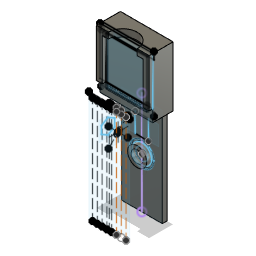
Variante Stifte Unten 20200217 v29 (Autodesk Fusion 360 archive; units mm, degrees)
design "Variante1"
Autodesk Fusion 360 part; units mm, degrees
mesh "Netz1" [no effect]
mesh "Netz2" [no effect]
sketch "Skizze1" plane through (0, 0, 0) normal (1, 0, 0) x (0, 0, -1)
  line L0 (1.7531, 23.1259) -> (1.7531, 20)
  line L1 (1.7531, 20) -> (-2.7469, 20)
  line L2 (-2.7469, 20) -> (-2.7469, -23)
  line L3 (-2.7469, -23) -> (-5.2469, -23)
  line L4 (-5.2469, -23) -> (-5.2469, 23.071)
  line L5 (1.7531, 23.071) -> (-5.2469, 23.071)
  dimension "d1" = 4.5
  dimension "d2" = 2.5
  dimension "d3" = 7.0002
  constraint vertical L0
  constraint perpendicular L0 L1
  constraint perpendicular L1 L2
  constraint perpendicular L2 L3
  constraint perpendicular L3 L4
  constraint coincident L0 L5.start
  constraint coincident L4 L5.end
  constraint perpendicular L4 L5
  measures "d1" distance of L0.end L1.end
  measures "d2" distance of L2.end L3.end
  measures "d3" distance of L0.start L4.end
extrude "Extrusion1" add sketch "Skizze1" along normal blind 8.5 makes body 1
extrude "Extrusion2" add 1 faces at (0, 22.0473, 2.0803) along direction (-1, 0, 0) blind 8.5 on bodies 1 bodies 1
sketch "Skizze2" plane through (0, 0, 2.7469) normal (0, 0, -1) x (-1, 0, 0)
  line L0 (8.5, 20) -> (-8.5, 20)
  line L1 (-8.5, 20) -> (-8.5, -23)
  line L2 (-8.5, -23) -> (8.5, -23)
  line L3 (8.5, -23) -> (8.5, 20)
  line L4 (2.8119, 12.0538) -> (-2.7881, 12.0538)
  line L5 (-2.7881, 12.0538) -> (-2.7881, 4.0538)
  line L6 (-2.7881, 4.0538) -> (2.8119, 4.0538)
  line L7 (2.8119, 4.0538) -> (2.8119, 12.0538)
  dimension "d8" = 5.6
  dimension "d9" = 8
  constraint horizontal L4
  constraint vertical L5
  constraint horizontal L6
  constraint vertical L7
  measures "d8" distance of L4.start L4.end
  measures "d9" distance of L4.start L6.end
extrude "Extrusion3" add sketch "Skizze2" along normal blind 8 contours L4 L5 L6 L7 bodies 1
sketch "Skizze3" plane through (-2.8119, 0, 0) normal (-1, 0, 0) x (0, 0, 1)
  line L0 (2.7469, 4.0538) -> (2.7469, 12.0538)
  line L1 (2.7469, 12.0538) -> (-5.2531, 12.0538)
  line L2 (-5.2531, 12.0538) -> (-5.2531, 4.0538)
  line L3 (-5.2531, 4.0538) -> (2.7469, 4.0538)
  line L4 (2.7469, 12.0538) -> (-5.2531, 4.0538) construction
  line L5 (2.7469, 4.0538) -> (-5.2531, 12.0538) construction
  circle A0 centre (-1.2531, 8.0538) radius 1.6
  line L6 (-5.2531, 8.0538) -> (-1.2531, 8.0538) construction
  line L7 (-1.2531, 8.0538) -> (2.7469, 8.0538) construction
  line L8 (-1.2531, 8.0538) -> (-1.2531, 12.0538) construction
  line L9 (-1.2531, 8.0538) -> (-1.2531, 4.0538) construction
  dimension "d12" = 3.2
  dimension "d13" = 8
  dimension "d14" = 8
  constraint coincident L0.end L1.start
  constraint coincident L2.end L3.start
  constraint coincident L0.start L3.end
  constraint coincident L1.end L2.start
  constraint midpoint L4 A0.centre
  constraint midpoint L2 L6.start
  constraint coincident A0.centre L6.end
  constraint midpoint L0 L7.end
  constraint midpoint L1 L8.end
  constraint midpoint L3 L9.end
  measures "d12" diameter of A0
  measures "d13" distance of L0 L2
  measures "d14" distance of L1.end L2.end
sketch "Skizze4" plane through (0, 0, 0) normal (1, 0, 0) x (0, 0, -1)
extrude "Extrusion4" add sketch "Skizze3" against normal blind 5.6 separate body makes body 2
sketch "Skizze5" plane through (0, 0, 2.7469) normal (0, 0, -1) x (-1, 0, 0)
  circle A0 centre (0, -1.9896) radius 2.4976 construction
  line L0 (0, 20) -> (0, -23) construction
  circle A1 centre (0, -1.9896) radius 2.5 construction
  circle A2 centre (0, -1.9896) radius 2.5
  circle A3 centre (0, -1.9896) radius 5
  circle A4 centre (0, -1.9896) radius 4
  dimension "d17" = 5
  dimension "d18" = 5
  dimension "d19" = 10
  dimension "d20" = 8
  constraint concentric A0 A1
  constraint concentric A1 A2
  constraint concentric A2 A3
  constraint concentric A1 A4
  measures "d17" diameter of A1
  measures "d18" diameter of A2
  measures "d19" diameter of A3
  measures "d20" diameter of A4
extrude "Extrusion5" add sketch "Skizze5" along normal blind 1 separate body contours A4 makes body 3
extrude "Extrusion6" add sketch "Skizze5" against normal blind 1 separate body contours A3 makes body 4
extrude "Extrusion7" cut sketch "Skizze5" against normal blind 1 contours A3 bodies 1 4
sketch "Skizze6" plane through (0, 0, 5.2469) normal (0, 0, 1) x (1, 0, 0)
  line L0 (-8.5, -23) -> (8.5, -23)
  line L1 (8.5, -23) -> (8.5, 23.071)
  line L2 (8.5, 23.071) -> (-8.5, 23.071)
  line L3 (-8.5, 23.071) -> (-8.5, -23)
  line L4 (-8.5, 23.071) -> (-8.5, 21.571) construction
  line L5 (-8.5, 21.571) -> (8.5, 21.571) construction
  line L6 (-8.5, 23.071) -> (0, 23.071) construction
  line L7 (0, 23.071) -> (0, -23) construction
  line L8 (0, 23.071) -> (1, 23.071) construction
  line L9 (1, 23.071) -> (3, 23.071) construction
  line L10 (3, 23.071) -> (5, 23.071) construction
  line L11 (0, 23.071) -> (-1, 23.071) construction
  line L12 (1, 23.071) -> (1, -23) construction
  line L13 (-1, 23.071) -> (-1, -23) construction
  line L14 (1, 23.071) -> (3, 23.071) construction
  line L15 (3, 23) -> (5, 23) construction
  line L16 (5, 23) -> (7, 23) construction
  line L17 (-1, 23.071) -> (-3, 23.071) construction
  line L18 (-3, 23.071) -> (-5, 23.071) construction
  line L19 (-5, 23.071) -> (-7, 23.071) construction
  line L20 (7, 23) -> (7, -23) construction
  line L21 (5, 23.071) -> (5, -23) construction
  line L22 (3, 23) -> (3, -23) construction
  line L23 (-3, 23.071) -> (-3, -23) construction
  line L24 (-5, 23.071) -> (-5, -23) construction
  line L25 (-7, 23.071) -> (-7, -23) construction
  circle A0 centre (7, 21.571) radius 0.5
  circle A1 centre (5, 21.571) radius 0.5
  circle A2 centre (3, 21.571) radius 0.5
  circle A3 centre (1, 21.571) radius 0.5
  circle A4 centre (-1, 21.571) radius 0.5
  circle A5 centre (-3, 21.571) radius 0.5
  circle A6 centre (-5, 21.571) radius 0.5
  circle A7 centre (-7, 21.571) radius 0.5
  point P0 (0, 23.071)
  dimension "d27" = 1.5
  dimension "d28" = 1
  dimension "d29" = 1
  dimension "d30" = 2
  dimension "d31" = 2
  dimension "d32" = 2
  dimension "d33" = 2
  dimension "d34" = 2
  dimension "d35" = 2
  dimension "d36" = 1
  dimension "d37" = 1
  dimension "d38" = 1
  dimension "d39" = 1
  dimension "d40" = 1
  dimension "d41" = 1
  dimension "d42" = 1
  dimension "d43" = 1
  constraint coincident L2.end L3.start
  constraint perpendicular L2 L4
  constraint coincident L1 L5.end
  constraint perpendicular L1 L5
  constraint coincident P0 L6.end
  constraint midpoint L0 L7.end
  constraint coincident L2 L8.end
  constraint coincident L2 L9.end
  constraint perpendicular L1 L9
  constraint coincident L2 L10.end
  constraint perpendicular L7 L11
  constraint coincident L0 L12.end
  constraint perpendicular L0 L12
  constraint coincident L0 L13.end
  constraint perpendicular L0 L13
  constraint perpendicular L12 L14
  constraint parallel L2 L15
  constraint parallel L15 L16
  constraint perpendicular L13 L17
  constraint parallel L2 L18
  constraint parallel L2 L19
  constraint coincident L0 L20.end
  constraint perpendicular L0 L20
  constraint perpendicular L10 L21
  constraint coincident L0 L22.end
  constraint perpendicular L0 L22
  constraint coincident L0 L23.end
  constraint perpendicular L0 L23
  constraint coincident L0 L24.end
  constraint perpendicular L0 L24
  constraint coincident L0 L25.end
  constraint perpendicular L0 L25
  constraint coincident L5 A0.centre
  constraint coincident L20 A0.centre
  constraint coincident L21 A1.centre
  constraint coincident L5 A1.centre
  constraint coincident L22 A2.centre
  constraint coincident L5 A2.centre
  constraint coincident L12 A3.centre
  constraint coincident L5 A3.centre
  constraint coincident L13 A4.centre
  constraint coincident L5 A4.centre
  constraint coincident L23 A5.centre
  constraint coincident L5 A5.centre
  constraint coincident L24 A6.centre
  constraint coincident L5 A6.centre
  constraint coincident L25 A7.centre
  constraint coincident L5 A7.centre
  measures "d27" distance of L2.end L4.end
  measures "d28" distance of P0 L8.end
  measures "d29" distance of P0 L11.end
  measures "d30" distance of L8.end L9.end
  measures "d31" distance of L15.start L15.end
  measures "d32" distance of L15.end L16.end
  measures "d33" distance of L11.end L17.end
  measures "d34" distance of L17.end L18.end
  measures "d35" distance of L18.end L19.end
  measures "d36" diameter of A0
  measures "d37" diameter of A1
  measures "d38" diameter of A2
  measures "d39" diameter of A3
  measures "d40" diameter of A4
  measures "d41" diameter of A5
  measures "d42" diameter of A6
  measures "d43" diameter of A7
hole "Bohrung1" at (7, 21.571, 5.2469) direction (0, 0, -1) diameter 1 depth 10 tip angle 118 bodies 1
hole "Bohrung2" at (5, 21.571, 5.2469) direction (0, 0, -1) diameter 1 depth 10 tip angle 118 bodies 1
hole "Bohrung3" at (3, 21.571, 5.2469) direction (0, 0, -1) diameter 1 depth 10 tip angle 118 bodies 1
hole "Bohrung4" at (1, 21.571, 5.2469) direction (0, 0, -1) diameter 1 depth 10 tip angle 118 bodies 1
hole "Bohrung5" at (-1, 21.571, 5.2469) direction (0, 0, -1) diameter 1 depth 10 tip angle 118 bodies 1
hole "Bohrung6" at (-3, 21.571, 5.2469) direction (0, 0, -1) diameter 1 depth 10 tip angle 118 bodies 1
hole "Bohrung7" at (-5, 21.571, 5.2469) direction (0, 0, -1) diameter 1 depth 10 tip angle 118 bodies 1
hole "Bohrung8" at (-7, 21.571, 5.2469) direction (0, 0, -1) diameter 1 depth 10 tip angle 118 bodies 1
extrude "Extrusion8" cut sketch "Skizze3" against normal blind 8.19 contours A0 bodies 1
sketch "Skizze7" plane through (0, 0, 0) normal (1, 0, 0) x (0, 0, -1)
  line L0 (10.3842, 40.5012) -> (2.3842, 40.5012)
  line L1 (2.3842, 40.5012) -> (2.3842, 20.0012)
  line L2 (2.3842, 20.0012) -> (8.3842, 20.0012)
  line L3 (8.3842, 20.0012) -> (8.3842, -22.9988)
  line L4 (10.3842, 40.5012) -> (10.3842, -23)
  line L5 (10.3842, -23) -> (8.3842, -22.9988)
  line L6 (8.3842, 20.0012) -> (10.3842, 20.0012)
  line L7 (8.3842, 12.102) -> (-2.6158, 12.102)
  line L8 (-2.6158, 12.102) -> (-2.6158, 4.002)
  line L9 (-2.6158, 4.002) -> (8.3842, 4.002)
  line L10 (8.3842, 4.002) -> (8.3842, 12.102)
  circle A0 centre (1.2604, 8.0508) radius 1.6
  dimension "d70" = 8
  dimension "d71" = 20.5
  dimension "d72" = 6
  dimension "d73" = 43
  dimension "d74" = 11
  dimension "d75" = 8.1
  dimension "d76" = 3.2
  constraint perpendicular L0 L1
  constraint perpendicular L1 L2
  constraint perpendicular L2 L3
  constraint perpendicular L0 L4
  constraint perpendicular L4 L6
  constraint coincident L3 L7.start
  constraint perpendicular L3 L7
  constraint perpendicular L7 L8
  constraint coincident L3 L9.end
  constraint perpendicular L3 L9
  measures "d70" distance of L0.start L0.end
  measures "d71" distance of L0.end L1.end
  measures "d72" distance of L1.end L2.end
  measures "d73" distance of L2.end L3.end
  measures "d74" distance of L7.start L7.end
  measures "d75" distance of L7.end L8.end
  measures "d76" diameter of A0
extrude "Extrusion9" add sketch "Skizze7" along normal blind 8.5 separate body contours L3 L4 L5 L6 L10 makes body 5
extrude "Extrusion10" add 1 faces at (0, 0.3344, -9.7175) along direction (-1, 0, 0) blind 8.5 on bodies 5 bodies 5
extrude "Extrusion11" add sketch "Skizze7" along normal blind 11 contours L0 L1 L2 L4 L6 bodies 4 5
extrude "Extrusion12" add sketch "Skizze7" against normal blind 11 contours L0 L1 L2 L4 L6 bodies 4
extrude "Extrusion13" add sketch "Skizze7" along normal blind 7 separate body contours L3 L7 L8 L9 L10 makes body 6
extrude "Extrusion14" add sketch "Skizze7" against normal blind 7 contours L3 L7 L8 L9 L10 bodies 6
sketch "Skizze8" plane through (0, 0, -8.3842) normal (0, 0, -1) x (-1, 0, 0)
  line L0 (7, 12.102) -> (-7, 12.102)
  line L1 (-7, 12.102) -> (-7, 4.002)
  line L2 (-7, 4.002) -> (7, 4.002)
  line L3 (7, 4.002) -> (7, 12.102)
  line L4 (2.8149, 12.102) -> (-2.788, 12.102)
  line L5 (-2.788, 12.102) -> (-2.788, 4.002)
  line L6 (-2.788, 4.002) -> (2.8149, 4.002)
  line L7 (2.8149, 4.002) -> (2.8149, 12.102)
  constraint horizontal L4
  constraint vertical L5
  constraint horizontal L6
  constraint vertical L7
  constraint coincident L2 L5.end
  constraint coincident L0 L4.start
extrude "Extrusion15" cut sketch "Skizze8" against normal blind 11 contours L0 L2 L4 L5 L6 L7 bodies 6 makes body 7 at (-7, 8.0516, -6.5429)
extrude "Extrusion16" cut 1 faces at (-2.8149, 8.0516, -6.5429) along direction (-1, 0, 0) blind 0.1 on bodies 7 bodies 7
extrude "Extrusion17" cut 1 faces at (2.788, 8.0516, -6.5429) along direction (1, 0, 0) blind 0.1 on bodies 6 bodies 6
hole "Bohrung9" at (7, 21.571, -2.3842) direction (0, 0, -1) diameter 1 depth 10 tip angle 118 bodies 4
hole "Bohrung10" at (5, 21.571, -2.3842) direction (0, 0, -1) diameter 1 depth 10 tip angle 118 bodies 4
hole "Bohrung11" at (3, 21.571, 5.2469) direction (0, 0, -1) diameter 1 depth 10 tip angle 118 bodies 4
hole "Bohrung12" at (1, 21.571, 5.2469) direction (0, 0, -1) diameter 1 depth 10 tip angle 118 bodies 4
hole "Bohrung13" at (3, 21.571, 5.2469) direction (0, 0, -1) diameter 1 depth 30 tip angle 118 bodies 4
hole "Bohrung14" at (1, 21.571, 5.2469) direction (0, 0, -1) diameter 1 depth 30 tip angle 118 bodies 4
hole "Bohrung15" at (-1, 21.571, 5.2469) direction (0, 0, -1) diameter 1 depth 30 tip angle 118 bodies 4
hole "Bohrung16" at (-3, 21.571, 5.2469) direction (0, 0, -1) diameter 1 depth 30 tip angle 118 bodies 4
hole "Bohrung17" at (-5, 21.571, 5.2469) direction (0, 0, -1) diameter 1 depth 30 tip angle 118 bodies 4
hole "Bohrung18" at (-7, 21.571, 5.2469) direction (0, 0, -1) diameter 1 depth 30 tip angle 118 bodies 4
sketch "Skizze9" plane through (0, 0, -2.3842) normal (0, 0, 1) x (1, 0, 0)
  circle A0 centre (-7, 21.571) radius 0.5
  circle A1 centre (-5, 21.571) radius 0.5
  circle A2 centre (-3, 21.571) radius 0.5
  circle A3 centre (-1, 21.571) radius 0.5
  circle A4 centre (1, 21.571) radius 0.5
  circle A5 centre (3, 21.571) radius 0.5
  circle A6 centre (5, 21.571) radius 0.5
  circle A7 centre (7, 21.571) radius 0.5
  line L0 (-11, 20.0012) -> (11, 20.0012)
  line L1 (11, 20.0012) -> (11, 40.5012)
  line L2 (11, 40.5012) -> (-11, 40.5012)
  line L3 (-11, 40.5012) -> (-11, 20.0012)
  line L4 (-11, 20.0012) -> (-11, 21.5512) construction
  line L5 (11, 20.0012) -> (11, 21.5512) construction
  line L6 (11, 21.5512) -> (-11, 21.5512) construction
  line L7 (11, 21.5512) -> (11, 20.5012) construction
  line L8 (-11, 21.5512) -> (-11, 20.5012) construction
  line L9 (-11, 20.5012) -> (11, 20.5012) construction
  line L10 (0, 20.5012) -> (8.5, 20.5012) construction
  line L11 (8.5, 20.5012) -> (-8.55, 20.5012)
  line L12 (-8.55, 20.5012) -> (-8.55, 40.5012)
  line L13 (-8.55, 40.5012) -> (8.5, 40.5012)
  line L14 (8.5, 40.5012) -> (8.5, 20.5012)
  line L15 (8.5, 40.5012) -> (-8.55, 40.5012)
  dimension "d125" = 1.55
  dimension "d126" = 1.55
  dimension "d127" = 1.05
  dimension "d128" = 1.05
  dimension "d129" = 8.5
  dimension "d130" = 17.05
  dimension "d131" = 20
  dimension "d134" = 20.5
  constraint coincident L0.start L3.end
  constraint perpendicular L0 L4
  constraint coincident L0.end L1.start
  constraint perpendicular L0 L5
  constraint perpendicular L6 L7
  constraint perpendicular L6 L8
  constraint midpoint L9 L10.start
  constraint perpendicular L1 L10
  constraint horizontal L11
  constraint vertical L12
  constraint horizontal L13
  constraint vertical L14
  measures "d125" distance of L0.start L4.end
  measures "d126" distance of L0.end L5.end
  measures "d127" distance of L5.end L7.end
  measures "d128" distance of L4.end L8.end
  measures "d129" distance of L10.start L10.end
  measures "d130" distance of L10.end L11.end
  measures "d131" distance of L10.end L13.end
  measures "d134" distance of L0 L2
extrude "Extrusion18" add 1 faces at (3.6667, 40.5012, -7.7175) along direction (0, 1, 0) blind 3 on bodies 4 bodies 4
extrude "Extrusion19" add 1 faces at (-2.8333, 20.0012, -4.3842) along direction (0, -1, 0) blind 1.5 on bodies 4 bodies 4
extrude "Extrusion20" add sketch "Skizze9" along normal blind 0.5 contours L0 L1 L2 L3 L11 L12 L14 bodies 4
extrude "Extrusion21" add 1 faces at (3.6667, 19.0012, -2.3842) along direction (0, 0, 1) blind 0.5 on bodies 4 bodies 4
sketch "Skizze10" plane through (0, 0, -2.3842) normal (0, 0, 1) x (1, 0, 0)
  circle A0 centre (7, 21.571) radius 0.5
  circle A1 centre (5, 21.571) radius 0.5
  circle A2 centre (3, 21.571) radius 0.5
  circle A3 centre (1, 21.571) radius 0.5
  circle A4 centre (-1, 21.571) radius 0.5
  circle A5 centre (-3, 21.571) radius 0.5
  circle A6 centre (-5, 21.571) radius 0.5
  circle A7 centre (-7, 21.571) radius 0.5
  line L0 (-11, 40.5012) -> (-8.55, 40.5012)
  line L1 (-8.55, 40.5012) -> (-8.55, 20.5012)
  line L2 (-8.55, 20.5012) -> (8.5, 20.5012)
  line L3 (8.5, 20.5012) -> (8.5, 40.5012)
  line L4 (8.5, 40.5012) -> (11, 40.5012)
  line L5 (11, 40.5012) -> (11, 43.5012)
  line L6 (11, 43.5012) -> (-11, 43.5012)
  line L7 (-11, 43.5012) -> (-11, 40.5012)
  line L8 (11, 43.5012) -> (-11, 43.5012)
  line L9 (-11, 43.5012) -> (-11, 40.5012)
  line L10 (-11, 40.5012) -> (11, 40.5012)
  line L11 (11, 40.5012) -> (11, 43.5012)
  constraint horizontal L8
  constraint vertical L9
  constraint horizontal L10
  constraint vertical L11
  constraint coincident L0.start L7.end
  constraint coincident L5.end L6.start
extrude "Extrusion22" add sketch "Skizze10" along normal blind 0.5 contours L0 L4 L5 L6 L7 L8 L9 L10 L11 bodies 4
extrude "Extrusion23" cut sketch "Skizze9" against normal blind 0.3 contours L2 L11 L12 L13 L14 L15 bodies 4
extrude "Extrusion24" cut 1 faces at (3.6667, 43.5012, -4.7175) along direction (0, -1, 0) blind 0.5 on bodies 4 bodies 4
extrude "Extrusion25" add 1 faces at (-2.8333, 18.5012, -4.0509) along direction (0, -1, 0) blind 0.5 on bodies 4 bodies 4
sketch "Skizze12" plane through (0, 0, -8.3842) normal (0, 0, 1) x (1, 0, 0)
  line L0 (8.5, 18.0012) -> (-8.5, 18.0012)
  line L1 (-8.5, 18.0012) -> (-8.5, -22.9988)
  line L2 (-8.5, -22.9988) -> (8.5, -22.9988)
  line L3 (8.5, -22.9988) -> (8.5, 18.0012)
  circle A0 centre (0, -2) radius 4
  line L4 (0, 20.0012) -> (0, -22.9988)
  circle A1 centre (0, -2) radius 5
  circle A2 centre (0, -2) radius 2.5
  dimension "d149" = 8
  dimension "d150" = 10
  dimension "d155" = 5
  constraint coincident A0.centre L4
  constraint concentric A0 A1
  constraint concentric A1 A2
  measures "d149" diameter of A0
  measures "d150" diameter of A1
  measures "d155" diameter of A2
extrude "Extrusion26" add sketch "Skizze12" along normal blind 2 contours A0 L4 A2 | A0 L4 A2 | L4 A2 | L4 A2 bodies 4
extrude "Extrusion27" cut sketch "Skizze12" against normal blind 0.8 contours A0 L4 A1 | A0 L4 A1 bodies 4
extrude "Extrusion28" cut sketch "Skizze12" along normal blind 2 contours L4 A2 | L4 A2 bodies 4
sketch "Skizze13" plane through (-7, 0, 0) normal (-1, 0, 0) x (0, 0, 1)
  circle A0 centre (-1.2604, 8.0508) radius 1.6
  line L0 (-8.3842, 12.102) -> (-8.3842, 4.002)
  line L1 (-8.3842, 4.002) -> (2.6158, 4.002)
  line L2 (2.6158, 4.002) -> (2.6158, 12.102)
  line L3 (2.6158, 12.102) -> (-8.3842, 12.102)
  line L4 (1.5065, 9.6531) -> (-1.2438, 11.2392)
  line L5 (-1.2438, 11.2392) -> (-3.9931, 9.6565)
  line L6 (-3.9931, 9.6565) -> (-3.9931, 6.48)
  line L7 (-3.9931, 6.48) -> (-1.2391, 4.8863)
  line L8 (-1.2391, 4.8863) -> (1.5052, 6.4776)
  line L9 (1.5052, 6.4776) -> (1.5065, 9.6531)
  constraint vertical L6
extrude "Extrusion29" cut sketch "Skizze13" against normal blind 2 contours L4 L5 L6 L7 L8 L9 bodies 7
sketch "Skizze14" plane through (7, 0, 0) normal (1, 0, 0) x (0, 0, -1)
  circle A0 centre (1.2604, 8.0508) radius 1.6
  line L0 (8.3842, 4.002) -> (8.3842, 12.102)
  line L1 (8.3842, 12.102) -> (-2.6158, 12.102)
  line L2 (-2.6158, 12.102) -> (-2.6158, 4.002)
  line L3 (-2.6158, 4.002) -> (8.3842, 4.002)
  circle A1 centre (1.2604, 8.0508) radius 3
  dimension "d160" = 6
  constraint concentric A0 A1
  measures "d160" diameter of A1
extrude "Extrusion30" cut sketch "Skizze14" against normal blind 2 contours A1 bodies 6
sketch "Skizze15" plane through (0, 0, -1.8842) normal (0, 0, 1) x (1, 0, 0)
  line L0 (-8.55, 40.5012) -> (8.5, 40.5012)
  line L1 (8.5, 40.5012) -> (8.5, 20.5012)
  line L2 (8.5, 20.5012) -> (-8.55, 20.5012)
  line L3 (-8.55, 20.5012) -> (-8.55, 40.5012)
  line L4 (11, 43.0012) -> (-11, 43.0012)
  line L5 (-11, 43.0012) -> (-11, 18.0012)
  line L6 (-11, 18.0012) -> (11, 18.0012)
  line L7 (11, 18.0012) -> (11, 43.0012)
  line L8 (-11, 43.0012) -> (11, 43.0012)
  line L9 (11, 43.0012) -> (11, 23.0012)
  line L10 (11, 23.0012) -> (-11, 23.0012)
  line L11 (-11, 23.0012) -> (-11, 43.0012)
  line L12 (8.5, 23.0012) -> (-8.55, 23.0012)
  line L13 (-8.55, 23.0012) -> (-8.55, 40.5012)
  line L14 (-8.55, 40.5012) -> (8.5, 40.5012)
  line L15 (8.5, 40.5012) -> (8.5, 23.0012)
  dimension "d163" = 20
  constraint horizontal L8
  constraint vertical L9
  constraint horizontal L10
  constraint vertical L11
  constraint coincident L4.end L5.start
  constraint horizontal L12
  constraint vertical L13
  constraint horizontal L14
  constraint vertical L15
  constraint coincident L0.start L3.end
  constraint coincident L10 L12.start
  constraint coincident L1 L12.start
  measures "d163" distance of L4.end L10.end
extrude "Extrusion32" add sketch "Skizze15" along normal blind 1.5 contours L0 L1 L3 L4 L5 L7 L8 L9 L10 L11 L13 L14 L15 bodies 4
extrude "Extrusion31" add sketch "Skizze15" along normal blind 1 contours L0 L1 L3 L4 L5 L7 L8 L9 L10 L11 L13 L14 L15 bodies 4
sketch "Skizze16" plane through (0, 43.0012, 0) normal (0, 1, 0) x (-1, 0, 0)
  line L0 (-11, -0.3842) -> (-11, -10.3842)
  line L1 (-11, -10.3842) -> (11, -10.3842)
  line L2 (11, -10.3842) -> (11, -0.3842)
  line L3 (11, -0.3842) -> (-11, -0.3842)
  circle A0 centre (0, -0.4007) radius 6
  dimension "d168" = 12
  measures "d168" diameter of A0
extrude "Extrusion33" cut sketch "Skizze16" against normal blind 3 contours L3 A0 picked at (1.145, -4.1251) bodies 4
hidden bodies 1 2 3 6 7
